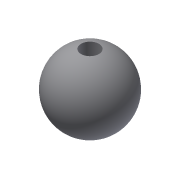
# Autodesk Inventor part: Ball Lever
Saved by Autodesk Inventor 2022 Beta2 (Build 260130000, 130) ContinuousBuild 0
## iProperties
Created: 2006-01-31
Part Number: Ball Lever
Document SubType Name: Modeling
Designer: landrews
Stock Number: Ball Lever
Density: 1 g/cm^3
Material: Generic
Mass: 10.8749 g
Surface Area: 28.0694 cm^2
Volume: 10.8749 cm^3
Appearance: Default
Author: landrews
Autodesk Inventor part; units mm, degrees
ref_plane "YZ Plane" through (0, 0, 0) normal (1, 0, 0) x (0, 1, 0)
ref_plane "XZ Plane" through (0, 0, 0) normal (0, 1, 0) x (-1, 0, 0)
sketch "Sketch2" plane through (0, 0, 0) normal (0, 1, 0) x (-1, 0, 0)
  line L0 (-22.4, 0) -> (16.8, 0) projected
  line L1 (0, -1.4) -> (0, 18.2) projected
  arc A0 (14, 0) -> (-14, 0) centre (0, 0) ccw
  dimension "d0" = 14
  constraints: 4 point on line, 2 point on circle, 1 centre point
  measures "d0" radius of A0
revolve "Revolution1" add sketch "Sketch2" angle 360 about axis through (0, 0, 0) along (-1, 0, 0)
ref_plane "Work Plane2" through (0, 0, 14) normal (0, 0, 1) x (1, 0, 0)
sketch "Sketch3" plane through (0, 0, 14) normal (0, 0, 1) x (1, 0, 0)
  point P0 (0, 0)
hole "Hole1" at (0, 0, 14) direction (0, 0, -1) diameter 6.917 depth 16 tip angle 118
body "Solid1"
